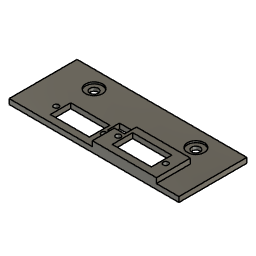
PlotClockServoHolder v2 (Autodesk Fusion 360 design; units mm, degrees)
Autodesk Fusion 360 part; units mm, degrees
sketch "Sketch1" plane through (0, 0, 0) normal (0, 0, 1) x (1, 0, 0)
  line L0 (50, 20) -> (-50, 20)
  line L1 (-50, 20) -> (-50, -20)
  line L2 (-50, -20) -> (50, -20)
  line L3 (50, -20) -> (50, 20)
  line L4 (50, 20) -> (-50, -20) construction
  line L5 (-50, 20) -> (50, -20) construction
  line L6 (35.75, -1) -> (-35.75, -1)
  line L7 (-35.75, -1) -> (-35.75, -19)
  line L8 (-35.75, -19) -> (35.75, -19)
  line L9 (35.75, -19) -> (35.75, -1)
  line L10 (35.75, -1) -> (-35.75, -19) construction
  line L11 (-35.75, -1) -> (35.75, -19) construction
  line L12 (-29.75, -4) -> (-29.75, -16)
  line L13 (29.75, -16) -> (29.75, -4)
  line L14 (29.75, -4) -> (-29.75, -16) construction
  line L15 (-29.75, -4) -> (29.75, -16) construction
  line L16 (-6.75, -16) -> (-6.75, -4)
  line L17 (6.75, -4) -> (6.75, -16)
  line L18 (6.75, -16) -> (-6.75, -4) construction
  line L19 (-6.75, -16) -> (6.75, -4) construction
  line L20 (29.75, -4) -> (6.75, -4)
  line L21 (-6.75, -4) -> (-29.75, -4)
  line L22 (-29.75, -16) -> (-6.75, -16)
  line L23 (6.75, -16) -> (29.75, -16)
  circle A0 centre (-32.25, -10) radius 1.5
  circle A1 centre (32.25, -10) radius 1.5
  circle A2 centre (-4.25, -10) radius 1.5
  circle A3 centre (4.25, -10) radius 1.5
  line L24 (0, -1) -> (0, -19)
  line L25 (5, 0) -> (-5, 0)
  line L26 (-5, 0) -> (-5, -7)
  line L27 (-5, -7) -> (5, -7)
  line L28 (5, -7) -> (5, 0)
  line L29 (5, 0) -> (-5, -7) construction
  line L30 (-5, 0) -> (5, -7) construction
  point P0 (0, -10)
  point P1 (0, -10)
  point P2 (0, -10)
  point P3 (-32.25, -10)
  point P4 (32.25, -10)
  point P5 (-4.25, -10)
  point P6 (4.25, -10)
  point P7 (0, -3.5)
  dimension "d1" = 100
  dimension "d2" = 40
  dimension "d3" = 71.5
  dimension "d4" = 18
  dimension "d5" = 1
  dimension "d6" = 59.5
  dimension "d7" = 12
  dimension "d8" = 13.5
  dimension "d9" = 12
  dimension "d10" = 3.5
  dimension "d11" = 3
  dimension "d12" = 3.5
  dimension "d13" = 3
  dimension "d14" = 2.5
  dimension "d15" = 2.5
  dimension "d16" = 3
  dimension "d17" = 3
  dimension "d44" = 10
  dimension "d45" = 7
  constraint horizontal L0
  constraint perpendicular L0 L1
  constraint parallel L0 L2
  constraint parallel L1 L3
  constraint coincident L4 origin
  constraint coincident L5 origin
  constraint horizontal L6
  constraint perpendicular L6 L7
  constraint parallel L6 L8
  constraint parallel L7 L9
  constraint coincident L10 P2
  constraint coincident L11 P2
  constraint vertical origin P2
  constraint horizontal L20
  constraint perpendicular L12 L20
  constraint parallel L20 L22
  constraint parallel L12 L13
  constraint coincident L14 P2
  constraint coincident L15 P2
  constraint coincident P2 P1
  constraint parallel L16 L17
  constraint coincident L18 P2
  constraint coincident L19 P2
  constraint collinear L20 L21
  constraint collinear L22 L23
  constraint coincident P3 A0.centre
  constraint coincident P4 A1.centre
  constraint coincident P5 A2.centre
  constraint coincident P6 A3.centre
  constraint midpoint L6 L24.start
  constraint midpoint L8 L24.end
  constraint horizontal L25
  constraint perpendicular L25 L26
  constraint parallel L25 L27
  constraint parallel L26 L28
  constraint coincident L29 P7
  constraint coincident L30 P7
  constraint coincident L24 P7
  constraint coincident origin L25
  measures "d1" distance of L1.end L2.end
  measures "d2" distance of L0.end L1.end
  measures "d3" distance of L7.end L8.end
  measures "d4" distance of L6.end L7.end
  measures "d5" distance of L2 L8
  measures "d6" distance of L12.end L13.start
  measures "d7" distance of L12.start L12.end
  measures "d8" distance of L16.end L17.start
  measures "d9" distance of L16.start L16.end
  measures "d10" distance of L7 P3
  measures "d11" diameter of A0
  measures "d12" distance of L9 P4
  measures "d13" diameter of A1
  measures "d14" distance of L16 P5
  measures "d15" distance of L17 P6
  measures "d16" diameter of A2
  measures "d17" diameter of A3
  measures "d44" distance of L26.end L27.end
  measures "d45" distance of L25.end L26.end
extrude "Extrude1" add sketch "Sketch1" along normal blind 3 contours L0 L1 L2 L3 | L6 L25 L26 L28 | L6 L24 L26 L27 | L6 L7 L8 L24 L26 L27 makes body 1
extrude "Extrude2" add sketch "Sketch1" along normal blind 6 and the other way blind -3 separate body contours L6 L8 L9 L24 L27 L28 | L6 L24 L27 L28 makes body 2
move_face "OffsetFaces1" offset 1 3 faces at (0, -7, 5) (23.8333, -1, 4) (35.75, -13, 5) on bodies 2
move_face "OffsetFaces2" offset 1 1 faces at (11.5833, -19, 5) on bodies 2
sketch "Sketch2" plane through (0, 0, 0) normal (0, 0, 1) x (1, 0, 0)
  line L0 (-50, 20) -> (-50, -20)
  line L1 (50, 20) -> (-50, 20)
  line L2 (50, -20) -> (50, 20)
  circle A0 centre (-30, 10) radius 2.5
  circle A1 centre (30, 10) radius 2.5
  circle A2 centre (-30, 10) radius 5
  circle A3 centre (30, 10) radius 5
  circle A4 centre (0, 10) radius 5
  circle A5 centre (0, 10) radius 2.5
  point P0 (-30, 10)
  point P1 (30, 10)
  dimension "d31" = 20
  dimension "d32" = 10
  dimension "d33" = 20
  dimension "d34" = 5
  dimension "d35" = 5
  dimension "d36" = 10
  dimension "d37" = 10
  dimension "d48" = 10
  dimension "d49" = 5
  constraint horizontal P0 A1.centre
  constraint coincident P0 A0.centre
  constraint coincident P1 A1.centre
  constraint concentric A1 A3
  constraint vertical origin A4.centre
  constraint horizontal P0 A4.centre
  constraint horizontal A4.centre A5.centre
  measures "d31" distance of P0 L0
  measures "d32" distance of P0 L1
  measures "d33" distance of P1 L2
  measures "d34" diameter of A0
  measures "d35" diameter of A1
  measures "d36" diameter of A2
  measures "d37" diameter of A3
  measures "d48" diameter of A4
  measures "d49" diameter of A5
extrude "Extrude3" cut sketch "Sketch2" along normal blind 3 contours A0 | A1 bodies 1
extrude "Extrude4" cut sketch "Sketch2" along normal blind 3 and the other way blind -2 contours A2 | A3 bodies 1
combine "Combine1" operation add target body 2 tool bodies 1
extrude "Extrude5" cut sketch "Sketch1" along normal blind 6 contours L6 L24 L27 L28 | L6 L25 L26 L28 | L6 L24 L26 L27 bodies 2
